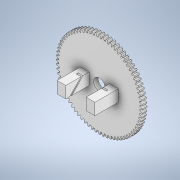
# Autodesk Inventor part: Gear-N72
Saved by Autodesk Inventor 2022.2 (Build 262287010, 287A)
## iProperties
CustomPartVersion: 1
Created: 2022-03-17
Part Number: Gear-N72
Material: Plástico ABS
Document SubType Name: Modeling
Designer: mabel
Categories: <?xml version="1.0" encoding="UTF-16"?> <MemberInstance><Categories><FamilyTemplate><FamilyTemplateParameter ValueType="xs:double" Id="1" ObjectReferenceKey="da_z" ObjectType="kUserParameterObject"/><FamilyTemplateParameter ValueType="xs:double" Id="2" ObjectReferenceKey="da_b" ObjectType="kUserParameterObject"/><FamilyTemplateParameter ValueType="xs:double" Id="3" ObjectReferenceKey="da_beta" ObjectType="kUserParameterObject"/><FamilyTemplateParameter ValueType="xs:double" Id="4" ObjectReferenceKey="da_da" ObjectType="kUserParameterObject"/><FamilyTemplateParameter ValueType="xs:double" Id="5" ObjectReferenceKey="da_aw" ObjectType="kUserParameterObject"/><FamilyTemplateParameter ValueType="xs:string" Id="6" ObjectReferenceKey="EAIAABAAAACIAQAAAAAAAIAAAAAAAAAA" ObjectType="83910656" SubObjectId="SurfaceGeometry"/></FamilyTemplate><ParamToTemplateMap><ParamToTemplate CategoryParameter="//CategoryParameter[@InternalName='046C89C9-8512-4d59-83FE-43B91F4F132A']" TemplateParameter="1"/><ParamToTemplate CategoryParameter="//CategoryParameter[@InternalName='2552DF32-E462-4b46-AEBF-C6C7768E72AC']" TemplateParameter="2"/><ParamToTemplate CategoryParameter="//CategoryParameter[@InternalName='C9EE641D-15FC-4fae-A226-E94C4372FDD7']" TemplateParameter="3"/><ParamToTemplate><ParamToTemplate CategoryParameter="//CategoryParameter[@InternalName='00B6519A-459B-49c7-AD84-2E56D39A5744']" ConstantValue="0.000000"/></ParamToTemplate><ParamToTemplate><ParamToTemplate CategoryParameter="//CategoryParameter[@InternalName='04B31F0E-C7A6-4894-AA32-9629BEFACF47']" ConstantValue="1.000000"/></ParamToTemplate><ParamToTemplate><ParamToTemplate CategoryParameter="//CategoryParameter[@InternalName='43CBEC2E-7847-49e7-A936-2F7889FCB2D9']" ConstantValue="0.250000"/></ParamToTemplate><ParamToTemplate><ParamToTemplate CategoryParameter="//CategoryParameter[@InternalName='B1EFC894-105D-4ebd-86BF-FA20ED196853']" ConstantValue="0.350000"/></ParamToTemplate><ParamToTemplate><ParamToTemplate CategoryParameter="//CategoryParameter[@InternalName='51175063-3D10-4879-93E8-6246FE8B403D']" ConstantValue="2060000000.000000"/></ParamToTemplate><ParamToTemplate><ParamToTemplate CategoryParameter="//CategoryParameter[@InternalName='A3A52E27-4454-46a9-B0BD-C932399B70AF']" ConstantValue="0.300000"/></ParamToTemplate><ParamToTemplate><ParamToTemplate CategoryParameter="//CategoryParameter[@InternalName='91B76062-C214-41d9-B1B9-14D2AB99603D']" ConstantValue="0.200000"/></ParamToTemplate><ParamToTemplate><ParamToTemplate CategoryParameter="//CategoryParameter[@InternalName='374E806E-8B8A-4dda-A9AA-1039D6500AD2']" ConstantValue="5.000000"/></ParamToTemplate><ParamToTemplate><ParamToTemplate CategoryParameter="//CategoryParameter[@InternalName='2D373A89-B862-43d6-8D0B-0CBF12AB9F6C']" ConstantValue="0.349066"/></ParamToTemplate><ParamToTemplate CategoryParameter="//CategoryParameter[@InternalName='37777632-D6A2-4fac-9D53-DB8ACD95C989']" TemplateParameter="4"/><ParamToTemplate CategoryParameter="//CategoryParameter[@InternalName='FD1017F1-B727-4f7e-9707-0F86F1FF9423']" TemplateParameter="5"/><ParamToTemplate><ParamToTemplate CategoryParameter="//CategoryParameter[@InternalName='9E1B4470-B2D3-4ff1-B813-535BB4CDF51A']" ConstantValue="3520000.000000"/></ParamToTemplate><ParamToTemplate><ParamToTemplate CategoryParameter="//CategoryParameter[@InternalName='F8452263-BFF6-458c-9FB1-07C4B99E95CD']" ConstantValue="11400000.000000"/></ParamToTemplate><ParamToTemplate><ParamToTemplate CategoryParameter="//CategoryParameter[@InternalName='3E3BB259-FD49-497f-8171-6EBC954A3479']" ConstantValue="2.000000"/></ParamToTemplate><ParamToTemplate CategoryParameter="//CategoryParameter[@InternalName='27C3BAF2-7550-4e4b-AE2C-0DB134B7D9B7']" TemplateParameter="6"/></ParamToTemplateMap><Category DisplayName="Gear" InternalName="DC85795E-93AB-48d5-8EEE-5A27447B64BD" Mnemonic="Gear"><CategoryParameter DisplayName="z" InternalName="046C89C9-8512-4d59-83FE-43B91F4F132A" Mnemonic="z"/><CategoryParameter DisplayName="b" InternalName="2552DF32-E462-4b46-AEBF-C6C7768E72AC" Mnemonic="b"/><CategoryParameter DisplayName="||b|" InternalName="C9EE641D-15FC-4fae-A226-E94C4372FDD7" Mnemonic="beta"/><CategoryParameter DisplayName="x" InternalName="00B6519A-459B-49c7-AD84-2E56D39A5744" Mnemonic="x"/><CategoryParameter DisplayName="a*" InternalName="04B31F0E-C7A6-4894-AA32-9629BEFACF47" Mnemonic="a"/><CategoryParameter DisplayName="c*" InternalName="43CBEC2E-7847-49e7-A936-2F7889FCB2D9" Mnemonic="c"/><CategoryParameter DisplayName="r|.f|*" InternalName="B1EFC894-105D-4ebd-86BF-FA20ED196853" Mnemonic="rf"/><CategoryParameter DisplayName="E" InternalName="51175063-3D10-4879-93E8-6246FE8B403D" Mnemonic="E"/><CategoryParameter DisplayName="||m|" InternalName="A3A52E27-4454-46a9-B0BD-C932399B70AF" Mnemonic="mi"/><Category DisplayName="SpurGear" InternalName="26C5A22E-A91E-4dfd-A3B3-23CCAFAE1764" Mnemonic="SpurGear"><CategoryParameter DisplayName="m" InternalName="91B76062-C214-41d9-B1B9-14D2AB99603D" Mnemonic="m"/><CategoryParameter DisplayName="P" InternalName="374E806E-8B8A-4dda-A9AA-1039D6500AD2" Mnemonic="PP"/><CategoryParameter DisplayName="||a|" InternalName="2D373A89-B862-43d6-8D0B-0CBF12AB9F6C" Mnemonic="alpha"/><CategoryParameter DisplayName="d|.a|" InternalName="37777632-D6A2-4fac-9D53-DB8ACD95C989" Mnemonic="da"/><CategoryParameter DisplayName="a|.w|" InternalName="FD1017F1-B727-4f7e-9707-0F86F1FF9423" Mnemonic="aw"/><CategoryParameter DisplayName="||s||.Flim|" InternalName="9E1B4470-B2D3-4ff1-B813-535BB4CDF51A" Mnemonic="sFlim"/><CategoryParameter DisplayName="||s||.Hlim|" InternalName="F8452263-BFF6-458c-9FB1-07C4B99E95CD" Mnemonic="sHlim"/><CategoryParameter DisplayName="tipo" InternalName="3E3BB259-FD49-497f-8171-6EBC954A3479" Mnemonic="type"/><CategoryParameter DisplayName="PitchDiameter" InternalName="27C3BAF2-7550-4e4b-AE2C-0DB134B7D9B7" Mnemonic="IDS_PITCHDIAM"/></Category></Category></Categories></MemberInstance>
Density: 1.06 g/cm^3
Appearance: Suave - Blanco
Author: mabel
Autodesk Inventor part; units mm, degrees
ref_plane "YZ Plane" through (0, 0, 0) normal (1, 0, 0) x (0, 1, 0)
ref_plane "XZ Plane" through (0, 0, 0) normal (0, 1, 0) x (-1, 0, 0)
ref_plane "XY Plane" through (0, 0, 0) normal (0, 0, 1) x (1, 0, 0)
sketch "Sketch1" plane through (0, 0, 0) normal (0, 0, 1) x (1, 0, 0)
  circle A0 centre (0, 0) radius 74
  dimension "d0" = 148
  constraints: 1 centre point
  measures "d0" diameter of A0
extrude "Extrusion1" add sketch "Sketch1" along normal blind 8
ref_plane "Work Plane2" through (0, 0, 4) normal (0, 0, 1) x (1, 0, 0)
sketch "Sketch2" plane through (0, 0, 0) normal (0, 0, -1) x (-1, 0, 0)
  circle A0 centre (0, 0) radius 74 projected
  circle A1 centre (0, 0) radius 72
  dimension "d3" = 144
  constraints: 1 centre point, 1 coincident
  measures "d3" diameter of A1
surface extrude "Diámetro de separación" sketch "Sketch2" against normal through all shown no curves A1
ref_plane "Work Plane8" through (0, 0, 0) normal (0.9990482, 0.0436194, 0) x (0, 0, 1)
ref_plane "Work Plane9" through (0, 0, 0) normal (1, 0, 0) x (0, 1, 0)
spur gear teeth "Engranaje recto" teeth 72 pitch diameter 144 tip diameter 148 root diameter 139 face width 15 start plane through (0, 0, 0) normal (0, 0, -1) x (-1, 0, 0)
sketch "Boceto3" plane through (0, 0, 8) normal (0, 0, 1) x (1, 0, 0)
  circle A0 centre (0, 0) radius 10
  dimension "d49" = 20
  constraints: 1 centre point, 1 coincident
  measures "d49" diameter of A0
extrude "Extrusión2" cut sketch "Boceto3" against normal through all
sketch "Boceto4" plane through (0, 0, 8) normal (0, 0, 1) x (1, 0, 0)
  arc A0 (-73.9956, 0.8072) -> (-73.9956, -0.8072) centre (0, 0) ccw construction
  line L0 (0, 0) -> (-25, 0) construction
  line L1 (-15, -10) -> (-30, -10)
  line L2 (-30, -10) -> (-30, 10)
  line L3 (-30, 10) -> (-15, 10)
  line L4 (-15, 10) -> (-15, -10)
  circle A1 centre (-25, 0) radius 0.75
  line L5 (-32, 10) -> (-22, -10) construction
  line L6 (-32, -10) -> (-22, 10) construction
  circle A2 centre (-27, 0) radius 0.0802
  dimension "d54" = 25
  dimension "d58" = 15
  dimension "d59" = 20
  dimension "d87" = 1.5
  constraints: 14 end point, 2 centre point, 2 horizontal, 2 parallel, 1 coincident, 1 midpoint, 1 perpendicular
  measures "d54" distance of L0.start L0.end
  measures "d58" distance of L2.end L3.end
  measures "d59" distance of L1.end L2.end
  measures "d87" diameter of A1
sketch "Boceto9" plane through (0, 0, 0) normal (0, 0, -1) x (-1, 0, 0)
  circle A0 centre (-40, 25) radius 2.5
  line L0 (-40, 25) -> (0, 25) construction
  line L1 (0, 0) -> (0, 25) construction
  dimension "d93" = 5
  dimension "d96" = 40
  dimension "d97" = 25
  constraints: 4 end point, 1 centre point, 1 horizontal, 1 vertical
  measures "d93" diameter of A0
  measures "d96" distance of L0.start L0.end
  measures "d97" distance of L1.start L0.end
extrude "Extrusión9" cut sketch "Boceto9" against normal blind 1
sketch "Boceto18" plane through (0, 0, 0) normal (0, 0, -1) x (-1, 0, 0)
  circle A0 centre (0, 0) radius 27.5 construction
  circle A1 centre (0, 0) radius 40 construction
  circle A2 centre (0, 0) radius 35 construction
  line L0 (0, 35) -> (0, 27.5) construction
  circle A3 centre (0, 31.25) radius 2.5
  line L1 (0, 0) -> (48.3926, 0) construction
  circle A4 centre (-31.25, 0) radius 2.5
  circle A5 centre (0, -31.25) radius 2.5
  circle A6 centre (31.25, 0) radius 2.5
  dimension "d113" = 55
  dimension "d115" = 70
  dimension "d114" = 80
  dimension "d116" = 5
  dimension "d119" = 360
  constraints: 5 centre point, 4 end point, 3 coincident, 2 vertical alignment, 1 horizontal, 1 midpoint, 1 vertical, 13 other
  measures "d114" diameter of A1
  measures "d116" diameter of A3
sketch "Boceto19" plane through (0, 0, 8) normal (0, 0, 1) x (1, 0, 0)
  line L0 (0, 0) -> (25, 0)
  line L1 (0, 0) -> (-25, 0)
  line L2 (-17.5, -10) -> (-32.5, -10)
  line L3 (-32.5, -10) -> (-32.5, 10)
  line L4 (-32.5, 10) -> (-17.5, 10)
  line L5 (-17.5, 10) -> (-17.5, -10)
  line L6 (-17.5, -10) -> (-32.5, 10) construction
  line L7 (-32.5, -10) -> (-17.5, 10) construction
  line L8 (32.5, -10) -> (17.5, -10)
  line L9 (17.5, -10) -> (17.5, 10)
  line L10 (17.5, 10) -> (32.5, 10)
  line L11 (32.5, 10) -> (32.5, -10)
  line L12 (58.3333, -10) -> (43.3333, 10) construction
  line L13 (43.3333, -10) -> (58.3333, 10) construction
  point P0 (50.8333, 0)
  dimension "d125" = 20
  dimension "d126" = 15
  dimension "d127" = 25
  dimension "d128" = 15
  dimension "d129" = 25
  constraints: 28 end point, 4 horizontal, 4 midpoint, 4 parallel, 2 perpendicular
  measures "d125" distance of L2.end L3.end
  measures "d126" distance of L3.end L4.end
  measures "d127" distance of L0.start L1.end
  measures "d128" distance of L9.end L10.end
  measures "d129" distance of L0.start L0.end
extrude "Extrusión14" add sketch "Boceto19" along normal blind 40
sketch "Boceto20" plane through (-17.5, -10, 8) normal (1, 0, 0) x (0, 0, -1)
  line L0 (0, 20) -> (0, 0) projected
  line L1 (-20, 0) -> (16.7696, 0) construction
  line L2 (0, 20) -> (-40, 20) projected
  line L3 (-24.2426, 0) -> (-20, 0)
  line L4 (0, 0) -> (-40, 0) projected
  line L5 (0, 0) -> (-30.5, 0)
  line L6 (0, 20) -> (-10.5, 20)
  line L7 (-30.5, 0) -> (-10.5, 20)
  line L8 (-10.5, 20) -> (-13.6, 20)
  line L9 (-30.5, 0) -> (-33.6, 0)
  line L10 (-33.6, 0) -> (-13.6, 20)
  point P0 (8, 10)
  point P1 (-40, 20)
  point P2 (-44.2426, 20)
  dimension "d134" = 30.5
  dimension "d135" = 10.5
  dimension "d136" = 3.1
  dimension "d137" = 3.1
  constraints: 16 end point, 6 point on line, 1 horizontal
  measures "d134" distance of L0.end L5.end
  measures "d135" distance of L0.start L6.end
  measures "d136" distance of L6.end L8.end
  measures "d137" distance of L5.end L9.end
extrude "Extrusión16" cut sketch "Boceto20" against normal blind 8 contours L7 L4 L10 L2
mirror "Simetría3" about plane through (0, 0, 0) normal (1, 0, 0) of "Extrusión16"
equation "\"d0\" = da_da"
equation "\"d3\" = da_d"
equation "\"da_da\" = 148"
equation "\"da_d\" = 144"
body "Solid1"
body "Srf1"
